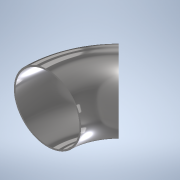
# Autodesk Inventor part: Kolano 45° ø85x2 R90
Saved by Autodesk Inventor 2020 (Build 240168000, 168)
## iProperties
RuleStatus: InUse
Created: 2021-10-14
Part Number: Kolano 45° ø85x2 R90
Material: 304L
Description: Kolano 45° ø85x2 R90
Document SubType Name: Modelowanie
Designer: inż. R.Jargiło
Density: 8 g/cm^3
Sheet Metal Rule: 1,5
Sheet Metal Width: 0,000 mm
Sheet Metal Length: 0,000 mm
Sheet Metal Area: 0,000 mm^2
Appearance: Częściowo polerowany(1)
Mass: 58.943 g
Surface Area: 91.7698 cm^2
Volume: 7.36788 cm^3
Project: 0479
Author: inż. R.Jargiło
Autodesk Inventor part; units mm, degrees
ref_plane "YZ Plane" through (0, 0, 0) normal (1, 0, 0) x (0, 1, 0)
ref_plane "XZ Plane" through (0, 0, 0) normal (0, 1, 0) x (-1, 0, 0)
sketch "Szkic6" plane through (0, 0, 0) normal (0, 0, 1) x (1, 0, 0)
  line L0 (-29.6067, 0) -> (35.2678, 0) construction
  line L1 (0, 42.3419) -> (0, -58.3726) construction
  arc A0 (26.3604, 0) -> (0, -63.6396) centre (90, -63.6396) ccw
  line L2 (0, -63.6396) -> (90, -63.6396) construction
  line L3 (90, -63.6396) -> (43.6611, -17.3007) construction
  line L4 (26.3604, 0) -> (26.3604, 0)
  line L5 (0, -63.6396) -> (0, -63.6396)
  point P0 (0, 0)
  dimension "d24" = 90
  dimension "d31" = 45
  dimension "d36" = 0
  dimension "d37" = 0
  constraints: 8 end point, 4 point on line, 2 point on circle, 1 centre point, 1 horizontal, 1 tangent, 1 vertical alignment
  measures "d24" radius of A0
  measures "d31" angle of L2 L3
  measures "d36" distance of L4.start L4.end
  measures "d37" distance of L2.start L5.end
ref_plane "Płaszczyzna konstrukcyjna2" through (0, -63.6396, 0) normal (0, -1, 0) x (1, 0, 0)
sketch "Szkic8" plane through (0, -63.6396, 0) normal (0, -1, 0) x (1, 0, 0)
  circle A0 centre (0, 0) radius 42.5
  circle A1 centre (0, 0) radius 40.5
  dimension "d32" = 85
  dimension "d33" = 2
  constraints: 2 centre point, 1 coincident
  measures "d32" diameter of A0
  measures "d33" radial gap between concentric circles of A0 A1
sweep "Przeciągnięcie2" add profiles "Szkic8" path "Szkic6"
equation "\"d32\" = OD"
equation "\"d33\" = THK"
equation "\"d24\" = R"
equation "\"d31\" = KAT"
equation "\"SzerokośćGięciaPodcięcia\" = Grubość"
equation "\"RozmiarPodcięciaNarożnika\" = 4 * Grubość"
equation "\"PromieńPrzejścia\" = PromieńGięcia"
equation "\"Rozmiar_promienia_Jacobiego\" = PromieńGięcia"
equation "\"Wielk_odstępu\" = Grubość"
equation "\"d2\" = PromieńGięcia"
equation "\"d23\" = PromieńGięcia"
equation "\"R\" = 90"
equation "\"OD\" = 85"
equation "\"THK\" = 2"
equation "\"KAT\" = 45deg"
equation "\"PROSTKA\" = 0"
equation "\"Grubość\" = 1.5"
equation "\"PromieńGięcia\" = 3"
